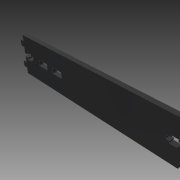
# Autodesk Inventor part: front_panel_2004_front
Saved by Autodesk Inventor 2014 (Build 180170000, 170)
## iProperties
Created: 2014-01-11
Part Number: front_panel_2004_front
Material: Generic
Document SubType Name: Modeling
Designer: buben
Density: 1 g/cm^3
Appearance: Anodized - Dark Gray
Author: buben
Autodesk Inventor part; units mm, degrees
ref_plane "YZ Plane" through (0, 0, 0) normal (1, 0, 0) x (0, 1, 0)
ref_plane "XZ Plane" through (0, 0, 0) normal (0, 1, 0) x (-1, 0, 0)
ref_plane "XY Plane" through (0, 0, 0) normal (0, 0, 1) x (1, 0, 0)
sketch "Sketch1" plane through (0, 0, 0) normal (0, 1, 0) x (-1, 0, 0)
  line L0 (0, 0) -> (220, 0)
  line L1 (220, 0) -> (220, 53.1)
  line L2 (220, 53.1) -> (0, 53.1)
  line L3 (0, 53.1) -> (0, 0)
  dimension "d0" = 53.1
  dimension "d1" = 220
  constraints: 8 end point, 2 parallel, 1 horizontal, 1 perpendicular
  measures "d0" distance of L2.end L0.start
  measures "d1" distance of L1.end L2.end
extrude "Extrusion1" add sketch "Sketch1" along normal blind 6
sketch "Sketch2" plane through (0, 6, 0) normal (0, 1, 0) x (1, 0, 0)
  line L0 (-220, 0) -> (-220, -53.1) projected
  line L1 (0, -53.1) -> (0, 0) projected
  line L2 (-220, -8.0055) -> (-224, -8.0055)
  line L3 (-226, -10.0055) -> (-226, -14.0055)
  line L4 (-224, -16.0055) -> (-220, -16.0055)
  line L5 (-220, -16.0055) -> (-220, -8.0055)
  line L6 (-220, -37.0945) -> (-224, -37.0945)
  line L7 (-226, -39.0945) -> (-226, -43.0945)
  line L8 (-224, -45.0945) -> (-220, -45.0945)
  line L9 (-220, -45.0945) -> (-220, -37.0945)
  line L10 (0, -8.0055) -> (4, -8.0055)
  line L11 (6, -10.0055) -> (6, -14.0055)
  line L12 (4, -16.0055) -> (0, -16.0055)
  line L13 (0, -16.0055) -> (0, -8.0055)
  line L14 (0, -37.0945) -> (4, -37.0945)
  line L15 (6, -39.0945) -> (6, -43.0945)
  line L16 (4, -45.0945) -> (0, -45.0945)
  line L17 (0, -45.0945) -> (0, -37.0945)
  arc A0 (-224, -8.0055) -> (-226, -10.0055) centre (-224, -10.0055) ccw
  arc A1 (-226, -14.0055) -> (-224, -16.0055) centre (-224, -14.0055) ccw
  arc A2 (-224, -37.0945) -> (-226, -39.0945) centre (-224, -39.0945) ccw
  arc A3 (-226, -43.0945) -> (-224, -45.0945) centre (-224, -43.0945) ccw
  arc A4 (4, -45.0945) -> (6, -43.0945) centre (4, -43.0945) ccw
  arc A5 (6, -39.0945) -> (4, -37.0945) centre (4, -39.0945) ccw
  arc A6 (4, -16.0055) -> (6, -14.0055) centre (4, -14.0055) ccw
  arc A7 (6, -10.0055) -> (4, -8.0055) centre (4, -10.0055) ccw
  line L18 (-222, -16.0055) -> (-222, -37.0945) construction
  point P0 (-222, -26.55)
  point P1 (-220, -26.55)
  dimension "d4" = 2
  dimension "d5" = 8
  dimension "d6" = 8
  dimension "d7" = 6
  dimension "d8" = 6
  dimension "d9" = 21.089
  constraints: 34 end point, 16 point on circle, 16 tangent, 8 centre point, 8 parallel, 7 equal radius, 6 collinear, 4 horizontal, 4 midpoint, 4 perpendicular, 4 point on line, 1 horizontal alignment
  measures "d4" radius of A0
  measures "d5" distance between parallel lines of L4 L2
  measures "d6" distance between parallel lines of L8 L6
  measures "d7" distance between parallel lines of L0 L3
  measures "d8" distance between parallel lines of L1 L11
  measures "d9" distance of L18.start L18.end
extrude "Extrusion2" add sketch "Sketch2" against normal blind 6
sketch "Sketch3" plane through (0, 6, 0) normal (0, 1, 0) x (1, 0, 0)
  line L0 (0, 0) -> (-220, 0) projected
  line L1 (-220, -16.0055) -> (-220, -37.0945) projected
  line L2 (-220, -53.1) -> (0, -53.1) projected
  line L3 (-203.7, -24.3) -> (-203.7, -28.8)
  line L4 (-220, -28.8) -> (-220, -24.3)
  line L5 (-215, -21.8) -> (-207.7, -21.8)
  line L6 (-207.7, -31.3) -> (-215, -31.3)
  line L7 (-220, -24.3) -> (-215, -24.3)
  line L8 (-207.7, -24.3) -> (-203.7, -24.3)
  line L9 (-203.7, -28.8) -> (-207.7, -28.8)
  line L10 (-215, -28.8) -> (-220, -28.8)
  line L11 (-207.7, -21.8) -> (-207.7, -24.3)
  line L12 (-207.7, -28.8) -> (-207.7, -31.3)
  line L13 (-215, -31.3) -> (-215, -28.8)
  line L14 (-215, -24.3) -> (-215, -21.8)
  line L15 (-110, 0) -> (-110, -53.1) construction
  line L16 (-16.3, -24.3) -> (-16.3, -28.8)
  line L17 (0, -28.8) -> (0, -24.3)
  line L18 (-5, -21.8) -> (-12.3, -21.8)
  line L19 (-12.3, -31.3) -> (-5, -31.3)
  line L20 (0, -24.3) -> (-5, -24.3)
  line L21 (-12.3, -24.3) -> (-16.3, -24.3)
  line L22 (-16.3, -28.8) -> (-12.3, -28.8)
  line L23 (-5, -28.8) -> (0, -28.8)
  line L24 (-12.3, -21.8) -> (-12.3, -24.3)
  line L25 (-12.3, -28.8) -> (-12.3, -31.3)
  line L26 (-5, -31.3) -> (-5, -28.8)
  line L27 (-5, -24.3) -> (-5, -21.8)
  point P0 (-203.7, -26.55)
  point P1 (-220, -26.55)
  point P2 (-16.3, -26.55)
  point P3 (0, -26.55)
  dimension "d12" = 4.5
  dimension "d13" = 2.5
  dimension "d14" = 2.5
  dimension "d15" = 5
  dimension "d16" = 4
  dimension "d17" = 7.3
  constraints: 50 end point, 14 symmetric about line, 10 parallel, 5 collinear, 4 midpoint, 4 perpendicular, 3 horizontal, 1 horizontal alignment
  measures "d12" distance of L3.start L3.end
  measures "d13" distance of L5.end L8.start
  measures "d14" distance of L9.end L6.start
  measures "d15" distance of L10.start L4.start
  measures "d16" distance of L3.end L9.end
  measures "d17" distance of L6.start L6.end
extrude "Extrusion3" cut sketch "Sketch3" against normal blind 6
sketch "Sketch4" plane through (0, 0, 0) normal (0, -1, 0) x (1, 0, 0)
  line L0 (-203.7, 28.8) -> (-203.7, 24.3) projected
  line L1 (-190.7, 30.55) -> (-177.7, 30.55)
  line L2 (-176.7, 29.55) -> (-176.7, 23.55)
  line L3 (-177.7, 22.55) -> (-190.7, 22.55)
  line L4 (-191.7, 23.55) -> (-191.7, 29.55)
  line L5 (-165.7, 30.55) -> (-152.7, 30.55)
  line L6 (-151.7, 29.55) -> (-151.7, 23.55)
  line L7 (-152.7, 22.55) -> (-165.7, 22.55)
  line L8 (-166.7, 23.55) -> (-166.7, 29.55)
  arc A0 (-190.7, 30.55) -> (-191.7, 29.55) centre (-190.7, 29.55) ccw
  arc A1 (-176.7, 29.55) -> (-177.7, 30.55) centre (-177.7, 29.55) ccw
  arc A2 (-177.7, 22.55) -> (-176.7, 23.55) centre (-177.7, 23.55) ccw
  arc A3 (-191.7, 23.55) -> (-190.7, 22.55) centre (-190.7, 23.55) ccw
  arc A4 (-165.7, 30.55) -> (-166.7, 29.55) centre (-165.7, 29.55) ccw
  arc A5 (-151.7, 29.55) -> (-152.7, 30.55) centre (-152.7, 29.55) ccw
  arc A6 (-152.7, 22.55) -> (-151.7, 23.55) centre (-152.7, 23.55) ccw
  arc A7 (-166.7, 23.55) -> (-165.7, 22.55) centre (-165.7, 23.55) ccw
  point P0 (-203.7, 26.55)
  point P1 (-191.7, 26.55)
  dimension "d20" = 1
  dimension "d21" = 15
  dimension "d22" = 15
  dimension "d23" = 8
  dimension "d24" = 10
  dimension "d25" = 12
  constraints: 16 end point, 16 point on circle, 16 tangent, 8 centre point, 7 equal radius, 4 parallel, 2 collinear, 2 horizontal, 2 midpoint, 2 perpendicular, 1 horizontal alignment
  measures "d20" radius of A0
  measures "d21" distance between parallel lines of L2 L4
  measures "d22" distance between parallel lines of L6 L8
  measures "d23" distance between parallel lines of L3 L1
  measures "d24" distance between parallel lines of L8 L2
  measures "d25" distance between parallel lines of L0 L4
extrude "Extrusion4" cut sketch "Sketch4" against normal through all
sketch "Sketch6" plane through (0, 6, 0) normal (0, 1, 0) x (1, 0, 0)
  line L0 (-220, -53.1) -> (0, -53.1) projected
  line L1 (0, -53.1) -> (0, -45.0945) projected
  line L2 (-50, -37.1) -> (-10, -37.1) construction
  line L3 (-10, -37.1) -> (-10, -47.1) construction
  line L4 (-10, -47.1) -> (-50, -47.1) construction
  line L5 (-50, -47.1) -> (-50, -37.1) construction
  spline S0 degree 2 poles (-43.1283, -39.4018) (-43.1283, -40.2833) (-43.8661, -40.7828) knots 0 0 0 1 1 1
  spline S1 degree 2 poles (-43.8661, -40.7828) (-44.16, -40.9787) (-44.5518, -40.9787) knots 0 0 0 1 1 1
  line L6 (-44.5518, -40.9787) -> (-45.9035, -40.9787)
  spline S2 degree 2 poles (-45.9035, -40.9787) (-46.07, -40.9787) (-46.07, -40.8514) knots 0 0 0 1 1 1
  spline S3 degree 2 poles (-46.07, -40.8514) (-46.07, -40.7273) (-45.9035, -40.7273) knots 0 0 0 1 1 1
  line L7 (-45.9035, -40.7273) -> (-45.6912, -40.7273)
  line L8 (-45.6912, -40.7273) -> (-45.6912, -37.7301)
  line L9 (-45.6912, -37.7301) -> (-45.9035, -37.7301)
  spline S4 degree 2 poles (-45.9035, -37.7301) (-46.07, -37.7301) (-46.07, -37.6028) knots 0 0 0 1 1 1
  spline S5 degree 2 poles (-46.07, -37.6028) (-46.07, -37.4787) (-45.9035, -37.4787) knots 0 0 0 1 1 1
  line L10 (-45.9035, -37.4787) -> (-44.5518, -37.4787)
  spline S6 degree 2 poles (-44.5518, -37.4787) (-43.9282, -37.4787) (-43.5723, -37.9097) knots 0 0 0 1 1 1
  spline S7 degree 2 poles (-43.5723, -37.9097) (-43.1283, -38.4484) (-43.1283, -39.0557) knots 0 0 0 1 1 1
  line L11 (-43.1283, -39.0557) -> (-43.1283, -39.4018)
  line L12 (-43.3797, -39.4573) -> (-43.3797, -39.0002)
  spline S8 degree 2 poles (-43.3797, -39.0002) (-43.3797, -38.7684) (-43.4548, -38.5855) knots 0 0 0 1 1 1
  spline S9 degree 2 poles (-43.4548, -38.5855) (-43.5625, -38.3178) (-43.7584, -38.0795) knots 0 0 0 1 1 1
  spline S10 degree 2 poles (-43.7584, -38.0795) (-44.0457, -37.7301) (-44.5289, -37.7301) knots 0 0 0 1 1 1
  line L13 (-44.5289, -37.7301) -> (-45.4398, -37.7301)
  line L14 (-45.4398, -37.7301) -> (-45.4398, -40.7273)
  line L15 (-45.4398, -40.7273) -> (-44.5289, -40.7273)
  spline S11 degree 2 poles (-44.5289, -40.7273) (-44.2155, -40.7273) (-43.9314, -40.5184) knots 0 0 0 1 1 1
  spline S12 degree 2 poles (-43.9314, -40.5184) (-43.6604, -40.3225) (-43.5168, -40.0254) knots 0 0 0 1 1 1
  spline S13 degree 2 poles (-43.5168, -40.0254) (-43.3797, -39.7381) (-43.3797, -39.4573) knots 0 0 0 1 1 1
  spline S14 degree 2 poles (-39.6642, -40.5674) (-39.6642, -40.6163) (-39.7132, -40.6686) knots 0 0 0 1 1 1
  spline S15 degree 2 poles (-39.7132, -40.6686) (-39.896, -40.8547) (-40.3041, -40.9755) knots 0 0 0 1 1 1
  spline S16 degree 2 poles (-40.3041, -40.9755) (-40.66, -41.0767) (-40.9734, -41.0767) knots 0 0 0 1 1 1
  spline S17 degree 2 poles (-40.9734, -41.0767) (-41.6035, -41.0767) (-42.0378, -40.6686) knots 0 0 0 1 1 1
  spline S18 degree 2 poles (-42.0378, -40.6686) (-42.4851, -40.2539) (-42.4851, -39.6303) knots 0 0 0 1 1 1
  spline S19 degree 2 poles (-42.4851, -39.6303) (-42.4851, -39.0557) (-42.0639, -38.6704) knots 0 0 0 1 1 1
  spline S20 degree 2 poles (-42.0639, -38.6704) (-41.6525, -38.2982) (-41.0779, -38.2982) knots 0 0 0 1 1 1
  spline S21 degree 2 poles (-41.0779, -38.2982) (-40.4445, -38.2982) (-39.6642, -39.1112) (-39.6707, -39.7446) knots 0 0 0 1 2 2 2
  line L16 (-39.6707, -39.7446) -> (-42.2304, -39.7446)
  spline S22 degree 2 poles (-42.2304, -39.7446) (-42.1651, -40.2409) (-41.4762, -40.8253) (-40.9734, -40.8253) knots 0 0 0 1 2 2 2
  spline S23 degree 2 poles (-40.9734, -40.8253) (-40.3139, -40.8253) (-39.8829, -40.489) knots 0 0 0 1 1 1
  spline S24 degree 2 poles (-39.8829, -40.489) (-39.8242, -40.4433) (-39.785, -40.4433) knots 0 0 0 1 1 1
  spline S25 degree 2 poles (-39.785, -40.4433) (-39.6642, -40.4433) (-39.6642, -40.5674) knots 0 0 0 1 1 1
  spline S26 degree 2 poles (-39.9254, -39.4899) (-40.0005, -39.0655) (-40.6437, -38.5529) (-41.0746, -38.5529) knots 0 0 0 1 2 2 2
  spline S27 degree 2 poles (-41.0746, -38.5529) (-41.5121, -38.5529) (-42.1488, -39.0622) (-42.2271, -39.4899) knots 0 0 0 1 2 2 2
  line L17 (-42.2271, -39.4899) -> (-39.9254, -39.4899)
  spline S28 degree 2 poles (-36.1348, -40.2572) (-36.1348, -40.6751) (-36.5527, -40.8971) knots 0 0 0 1 1 1
  spline S29 degree 2 poles (-36.5527, -40.8971) (-36.8923, -41.0767) (-37.3461, -41.0767) knots 0 0 0 1 1 1
  spline S30 degree 2 poles (-37.3461, -41.0767) (-37.9403, -41.0767) (-38.319, -40.7763) knots 0 0 0 1 1 1
  spline S31 degree 2 poles (-38.319, -40.7763) (-38.319, -40.9232) (-38.3713, -40.9591) knots 0 0 0 1 1 1
  spline S32 degree 2 poles (-38.3713, -40.9591) (-38.4072, -40.9787) (-38.4431, -40.9787) knots 0 0 0 1 1 1
  spline S33 degree 2 poles (-38.4431, -40.9787) (-38.5704, -40.9787) (-38.5704, -40.8122) knots 0 0 0 1 1 1
  line L18 (-38.5704, -40.8122) -> (-38.5704, -40.2931)
  spline S34 degree 2 poles (-38.5704, -40.2931) (-38.5704, -40.1266) (-38.4431, -40.1266) knots 0 0 0 1 1 1
  spline S35 degree 2 poles (-38.4431, -40.1266) (-38.3158, -40.1266) (-38.3158, -40.2637) knots 0 0 0 1 1 1
  spline S36 degree 2 poles (-38.3158, -40.2637) (-38.3158, -40.5641) (-37.9109, -40.7306) knots 0 0 0 1 1 1
  spline S37 degree 2 poles (-37.9109, -40.7306) (-37.6856, -40.8253) (-37.3526, -40.8253) knots 0 0 0 1 1 1
  spline S38 degree 2 poles (-37.3526, -40.8253) (-37.0163, -40.8253) (-36.7486, -40.7077) knots 0 0 0 1 1 1
  spline S39 degree 2 poles (-36.7486, -40.7077) (-36.3862, -40.5543) (-36.3862, -40.2572) knots 0 0 0 1 1 1
  spline S40 degree 2 poles (-36.3862, -40.2572) (-36.3862, -39.7936) (-37.3396, -39.6956) knots 0 0 0 1 1 1
  spline S41 degree 2 poles (-37.3396, -39.6956) (-37.715, -39.6564) (-37.8783, -39.6107) knots 0 0 0 1 1 1
  spline S42 degree 2 poles (-37.8783, -39.6107) (-38.1884, -39.5258) (-38.3288, -39.3365) knots 0 0 0 1 1 1
  spline S43 degree 2 poles (-38.3288, -39.3365) (-38.4431, -39.1798) (-38.4431, -39.0002) knots 0 0 0 1 1 1
  spline S44 degree 2 poles (-38.4431, -39.0002) (-38.4431, -38.6443) (-38.0644, -38.4517) knots 0 0 0 1 1 1
  spline S45 degree 2 poles (-38.0644, -38.4517) (-37.7607, -38.2982) (-37.3689, -38.2982) knots 0 0 0 1 1 1
  spline S46 degree 2 poles (-37.3689, -38.2982) (-36.8498, -38.2982) (-36.5233, -38.5496) knots 0 0 0 1 1 1
  spline S47 degree 2 poles (-36.5233, -38.5496) (-36.5233, -38.3864) (-36.396, -38.3864) knots 0 0 0 1 1 1
  spline S48 degree 2 poles (-36.396, -38.3864) (-36.2687, -38.3864) (-36.2687, -38.5562) knots 0 0 0 1 1 1
  line L19 (-36.2687, -38.5562) -> (-36.2687, -38.9904)
  spline S49 degree 2 poles (-36.2687, -38.9904) (-36.2687, -39.1569) (-36.396, -39.1569) knots 0 0 0 1 1 1
  spline S50 degree 2 poles (-36.396, -39.1569) (-36.5103, -39.1569) (-36.5233, -39.0165) knots 0 0 0 1 1 1
  spline S51 degree 2 poles (-36.5233, -39.0165) (-36.5396, -38.8369) (-36.7094, -38.7194) knots 0 0 0 1 1 1
  spline S52 degree 2 poles (-36.7094, -38.7194) (-36.951, -38.5529) (-37.3559, -38.5529) knots 0 0 0 1 1 1
  spline S53 degree 2 poles (-37.3559, -38.5529) (-37.7803, -38.5529) (-38.0121, -38.7227) knots 0 0 0 1 1 1
  spline S54 degree 2 poles (-38.0121, -38.7227) (-38.1884, -38.8533) (-38.1884, -39.01) knots 0 0 0 1 1 1
  spline S55 degree 2 poles (-38.1884, -39.01) (-38.1884, -39.1896) (-37.9795, -39.3104) knots 0 0 0 1 1 1
  spline S56 degree 2 poles (-37.9795, -39.3104) (-37.8326, -39.392) (-37.4342, -39.4377) knots 0 0 0 1 1 1
  spline S57 degree 2 poles (-37.4342, -39.4377) (-36.9053, -39.4965) (-36.7094, -39.565) knots 0 0 0 1 1 1
  spline S58 degree 2 poles (-36.7094, -39.565) (-36.1348, -39.774) (-36.1348, -40.2572) knots 0 0 0 1 1 1
  spline S59 degree 2 poles (-32.3867, -40.8514) (-32.3867, -40.9787) (-32.5564, -40.9787) knots 0 0 0 1 1 1
  line L20 (-32.5564, -40.9787) -> (-34.7831, -40.9787)
  spline S60 degree 2 poles (-34.7831, -40.9787) (-34.9496, -40.9787) (-34.9496, -40.8514) knots 0 0 0 1 1 1
  spline S61 degree 2 poles (-34.9496, -40.8514) (-34.9496, -40.7273) (-34.7831, -40.7273) knots 0 0 0 1 1 1
  line L21 (-34.7831, -40.7273) -> (-33.7938, -40.7273)
  line L22 (-33.7938, -40.7273) -> (-33.7938, -38.6443)
  line L23 (-33.7938, -38.6443) -> (-34.5285, -38.6443)
  spline S62 degree 2 poles (-34.5285, -38.6443) (-34.6982, -38.6443) (-34.6982, -38.517) knots 0 0 0 1 1 1
  spline S63 degree 2 poles (-34.6982, -38.517) (-34.6982, -38.3896) (-34.5285, -38.3896) knots 0 0 0 1 1 1
  line L24 (-34.5285, -38.3896) -> (-33.5424, -38.3896)
  line L25 (-33.5424, -38.3896) -> (-33.5424, -40.7273)
  line L26 (-33.5424, -40.7273) -> (-32.5564, -40.7273)
  spline S64 degree 2 poles (-32.5564, -40.7273) (-32.3867, -40.7273) (-32.3867, -40.8514) knots 0 0 0 1 1 1
  line L27 (-33.549, -37.7497) -> (-33.9212, -37.7497)
  line L28 (-33.9212, -37.7497) -> (-33.9212, -37.1)
  line L29 (-33.9212, -37.1) -> (-33.549, -37.1)
  line L30 (-33.549, -37.1) -> (-33.549, -37.7497)
  spline S65 degree 2 poles (-28.3969, -38.517) (-28.3969, -38.6443) (-28.5634, -38.6443) knots 0 0 0 1 1 1
  line L31 (-28.5634, -38.6443) -> (-28.903, -38.6443)
  line L32 (-28.903, -38.6443) -> (-28.903, -41.1518)
  spline S66 degree 2 poles (-28.903, -41.1518) (-28.903, -41.4032) (-29.0107, -41.5991) knots 0 0 0 1 1 1
  spline S67 degree 2 poles (-29.0107, -41.5991) (-29.1772, -41.906) (-29.556, -42.0725) knots 0 0 0 1 1 1
  spline S68 degree 2 poles (-29.556, -42.0725) (-29.6931, -42.1313) (-29.9249, -42.1313) knots 0 0 0 1 1 1
  line L33 (-29.9249, -42.1313) -> (-30.6367, -42.1313)
  spline S69 degree 2 poles (-30.6367, -42.1313) (-30.8032, -42.1313) (-30.8032, -42.0039) knots 0 0 0 1 1 1
  spline S70 degree 2 poles (-30.8032, -42.0039) (-30.8032, -41.8766) (-30.6367, -41.8766) knots 0 0 0 1 1 1
  line L34 (-30.6367, -41.8766) -> (-29.9151, -41.8799)
  spline S71 degree 2 poles (-29.9151, -41.8799) (-29.458, -41.8831) (-29.2197, -41.4358) knots 0 0 0 1 1 1
  spline S72 degree 2 poles (-29.2197, -41.4358) (-29.1544, -41.3118) (-29.1544, -41.1159) knots 0 0 0 1 1 1
  line L35 (-29.1544, -41.1159) -> (-29.1544, -40.3617)
  spline S73 degree 2 poles (-29.1544, -40.3617) (-29.5592, -40.9167) (-30.1959, -40.9167) knots 0 0 0 1 1 1
  spline S74 degree 2 poles (-30.1959, -40.9167) (-30.7281, -40.9167) (-31.097, -40.5249) knots 0 0 0 1 1 1
  spline S75 degree 2 poles (-31.097, -40.5249) (-31.4627, -40.1429) (-31.4627, -39.6075) knots 0 0 0 1 1 1
  spline S76 degree 2 poles (-31.4627, -39.6075) (-31.4627, -39.0688) (-30.7281, -38.2982) (-30.1959, -38.2982) knots 0 0 0 1 2 2 2
  spline S77 degree 2 poles (-30.1959, -38.2982) (-29.5592, -38.2982) (-29.1544, -38.85) knots 0 0 0 1 1 1
  line L36 (-29.1544, -38.85) -> (-29.1544, -38.3896)
  line L37 (-29.1544, -38.3896) -> (-28.5634, -38.3896)
  spline S78 degree 2 poles (-28.5634, -38.3896) (-28.3969, -38.3896) (-28.3969, -38.517) knots 0 0 0 1 1 1
  spline S79 degree 2 poles (-29.1544, -39.6075) (-29.1544, -39.17) (-29.7486, -38.5529) (-30.1828, -38.5529) knots 0 0 0 1 2 2 2
  spline S80 degree 2 poles (-30.1828, -38.5529) (-30.6171, -38.5529) (-31.208, -39.1732) (-31.208, -39.6075) knots 0 0 0 1 2 2 2
  spline S81 degree 2 poles (-31.208, -39.6075) (-31.208, -40.0417) (-30.6171, -40.662) (-30.1828, -40.662) knots 0 0 0 1 2 2 2
  spline S82 degree 2 poles (-30.1828, -40.662) (-29.7486, -40.662) (-29.1544, -40.0417) (-29.1544, -39.6075) knots 0 0 0 1 2 2 2
  spline S83 degree 2 poles (-24.8414, -40.8514) (-24.8414, -40.9787) (-25.0079, -40.9787) knots 0 0 0 1 1 1
  line L38 (-25.0079, -40.9787) -> (-25.6805, -40.9787)
  spline S84 degree 2 poles (-25.6805, -40.9787) (-25.8503, -40.9787) (-25.8503, -40.8514) knots 0 0 0 1 1 1
  spline S85 degree 2 poles (-25.8503, -40.8514) (-25.8503, -40.7273) (-25.6805, -40.7273) knots 0 0 0 1 1 1
  line L39 (-25.6805, -40.7273) -> (-25.4715, -40.7273)
  line L40 (-25.4715, -40.7273) -> (-25.4715, -39.1863)
  spline S86 degree 2 poles (-25.4715, -39.1863) (-25.4715, -38.8924) (-25.687, -38.7161) knots 0 0 0 1 1 1
  spline S87 degree 2 poles (-25.687, -38.7161) (-25.8862, -38.5529) (-26.1866, -38.5529) knots 0 0 0 1 1 1
  spline S88 degree 2 poles (-26.1866, -38.5529) (-26.4902, -38.5529) (-26.7285, -38.7292) knots 0 0 0 1 1 1
  spline S89 degree 2 poles (-26.7285, -38.7292) (-26.8657, -38.8304) (-27.1367, -39.1504) knots 0 0 0 1 1 1
  line L41 (-27.1367, -39.1504) -> (-27.1367, -40.7273)
  line L42 (-27.1367, -40.7273) -> (-26.8526, -40.7273)
  spline S90 degree 2 poles (-26.8526, -40.7273) (-26.6861, -40.7273) (-26.6861, -40.8514) knots 0 0 0 1 1 1
  spline S91 degree 2 poles (-26.6861, -40.8514) (-26.6861, -40.9787) (-26.8526, -40.9787) knots 0 0 0 1 1 1
  line L43 (-26.8526, -40.9787) -> (-27.6721, -40.9787)
  spline S92 degree 2 poles (-27.6721, -40.9787) (-27.8386, -40.9787) (-27.8386, -40.8514) knots 0 0 0 1 1 1
  spline S93 degree 2 poles (-27.8386, -40.8514) (-27.8386, -40.7273) (-27.6721, -40.7273) knots 0 0 0 1 1 1
  line L44 (-27.6721, -40.7273) -> (-27.3881, -40.7273)
  line L45 (-27.3881, -40.7273) -> (-27.3881, -38.6443)
  line L46 (-27.3881, -38.6443) -> (-27.6003, -38.6443)
  spline S94 degree 2 poles (-27.6003, -38.6443) (-27.7668, -38.6443) (-27.7668, -38.517) knots 0 0 0 1 1 1
  spline S95 degree 2 poles (-27.7668, -38.517) (-27.7668, -38.3896) (-27.6003, -38.3896) knots 0 0 0 1 1 1
  line L47 (-27.6003, -38.3896) -> (-27.1367, -38.3896)
  line L48 (-27.1367, -38.3896) -> (-27.1367, -38.7684)
  spline S96 degree 2 poles (-27.1367, -38.7684) (-26.673, -38.2982) (-26.1833, -38.2982) knots 0 0 0 1 1 1
  spline S97 degree 2 poles (-26.1833, -38.2982) (-25.6283, -38.2982) (-25.354, -38.7161) knots 0 0 0 1 1 1
  spline S98 degree 2 poles (-25.354, -38.7161) (-25.2201, -38.9251) (-25.2201, -39.1438) knots 0 0 0 1 1 1
  line L49 (-25.2201, -39.1438) -> (-25.2201, -40.7273)
  line L50 (-25.2201, -40.7273) -> (-25.0079, -40.7273)
  spline S99 degree 2 poles (-25.0079, -40.7273) (-24.8414, -40.7273) (-24.8414, -40.8514) knots 0 0 0 1 1 1
  spline S100 degree 2 poles (-17.4855, -39.676) (-17.4855, -40.2441) (-17.8643, -40.6555) knots 0 0 0 1 1 1
  spline S101 degree 2 poles (-17.8643, -40.6555) (-18.2528, -41.0767) (-18.8209, -41.0767) knots 0 0 0 1 1 1
  spline S102 degree 2 poles (-18.8209, -41.0767) (-19.4771, -41.0767) (-19.9179, -40.4857) knots 0 0 0 1 1 1
  line L51 (-19.9179, -40.4857) -> (-19.9179, -40.9787)
  line L52 (-19.9179, -40.9787) -> (-20.5089, -40.9787)
  spline S103 degree 2 poles (-20.5089, -40.9787) (-20.6754, -40.9787) (-20.6754, -40.8514) knots 0 0 0 1 1 1
  spline S104 degree 2 poles (-20.6754, -40.8514) (-20.6754, -40.7273) (-20.5089, -40.7273) knots 0 0 0 1 1 1
  line L53 (-20.5089, -40.7273) -> (-20.1693, -40.7273)
  line L54 (-20.1693, -40.7273) -> (-20.1693, -37.4787)
  line L55 (-20.1693, -37.4787) -> (-20.5089, -37.4787)
  spline S105 degree 2 poles (-20.5089, -37.4787) (-20.6754, -37.4787) (-20.6754, -37.3514) knots 0 0 0 1 1 1
  spline S106 degree 2 poles (-20.6754, -37.3514) (-20.6754, -37.2241) (-20.5089, -37.2241) knots 0 0 0 1 1 1
  line L56 (-20.5089, -37.2241) -> (-19.9179, -37.2241)
  line L57 (-19.9179, -37.2241) -> (-19.9179, -38.8892)
  spline S107 degree 2 poles (-19.9179, -38.8892) (-19.4641, -38.2982) (-18.8209, -38.2982) knots 0 0 0 1 1 1
  spline S108 degree 2 poles (-18.8209, -38.2982) (-18.2528, -38.2982) (-17.4855, -39.1047) (-17.4855, -39.676) knots 0 0 0 1 2 2 2
  spline S109 degree 2 poles (-17.7369, -39.6891) (-17.7369, -39.2287) (-18.0471, -38.8924) knots 0 0 0 1 1 1
  spline S110 degree 2 poles (-18.0471, -38.8924) (-18.3671, -38.5529) (-18.8242, -38.5529) knots 0 0 0 1 1 1
  spline S111 degree 2 poles (-18.8242, -38.5529) (-19.2845, -38.5529) (-19.9146, -39.2287) (-19.9146, -39.6891) knots 0 0 0 1 2 2 2
  spline S112 degree 2 poles (-19.9146, -39.6891) (-19.9146, -40.1494) (-19.2845, -40.8253) (-18.8242, -40.8253) knots 0 0 0 1 2 2 2
  spline S113 degree 2 poles (-18.8242, -40.8253) (-18.3671, -40.8253) (-18.0471, -40.4857) knots 0 0 0 1 1 1
  spline S114 degree 2 poles (-18.0471, -40.4857) (-17.7369, -40.1494) (-17.7369, -39.6891) knots 0 0 0 1 1 1
  spline S115 degree 2 poles (-13.6199, -38.517) (-13.6199, -38.6051) (-13.6982, -38.6313) knots 0 0 0 1 1 1
  spline S116 degree 2 poles (-13.6982, -38.6313) (-13.7276, -38.6443) (-13.8647, -38.6443) knots 0 0 0 1 1 1
  line L58 (-13.8647, -38.6443) -> (-15.4515, -41.8799)
  line L59 (-15.4515, -41.8799) -> (-15.0597, -41.8799)
  spline S117 degree 2 poles (-15.0597, -41.8799) (-14.8932, -41.8799) (-14.8932, -42.0039) knots 0 0 0 1 1 1
  spline S118 degree 2 poles (-14.8932, -42.0039) (-14.8932, -42.1313) (-15.0597, -42.1313) knots 0 0 0 1 1 1
  line L60 (-15.0597, -42.1313) -> (-16.5093, -42.1313)
  spline S119 degree 2 poles (-16.5093, -42.1313) (-16.6758, -42.1313) (-16.6758, -42.0039) knots 0 0 0 1 1 1
  spline S120 degree 2 poles (-16.6758, -42.0039) (-16.6758, -41.8799) (-16.5093, -41.8799) knots 0 0 0 1 1 1
  line L61 (-16.5093, -41.8799) -> (-15.7225, -41.8799)
  line L62 (-15.7225, -41.8799) -> (-15.2785, -40.9787)
  line L63 (-15.2785, -40.9787) -> (-16.4473, -38.6443)
  line L64 (-16.4473, -38.6443) -> (-16.5224, -38.6443)
  spline S121 degree 2 poles (-16.5224, -38.6443) (-16.6889, -38.6443) (-16.6889, -38.517) knots 0 0 0 1 1 1
  spline S122 degree 2 poles (-16.6889, -38.517) (-16.6889, -38.4354) (-16.6171, -38.4027) knots 0 0 0 1 1 1
  spline S123 degree 2 poles (-16.6171, -38.4027) (-16.5877, -38.3896) (-16.5224, -38.3896) knots 0 0 0 1 1 1
  line L65 (-16.5224, -38.3896) -> (-15.8335, -38.3896)
  spline S124 degree 2 poles (-15.8335, -38.3896) (-15.667, -38.3896) (-15.667, -38.517) knots 0 0 0 1 1 1
  spline S125 degree 2 poles (-15.667, -38.517) (-15.667, -38.6443) (-15.8335, -38.6443) knots 0 0 0 1 1 1
  line L66 (-15.8335, -38.6443) -> (-16.173, -38.6443)
  line L67 (-16.173, -38.6443) -> (-15.1413, -40.7012)
  line L68 (-15.1413, -40.7012) -> (-14.1357, -38.6443)
  line L69 (-14.1357, -38.6443) -> (-14.4753, -38.6443)
  spline S126 degree 2 poles (-14.4753, -38.6443) (-14.6418, -38.6443) (-14.6418, -38.517) knots 0 0 0 1 1 1
  spline S127 degree 2 poles (-14.6418, -38.517) (-14.6418, -38.3896) (-14.4753, -38.3896) knots 0 0 0 1 1 1
  line L70 (-14.4753, -38.3896) -> (-13.7896, -38.3896)
  spline S128 degree 2 poles (-13.7896, -38.3896) (-13.6199, -38.3896) (-13.6199, -38.517) knots 0 0 0 1 1 1
  spline S129 degree 2 poles (-47.2257, -46.6443) (-47.2257, -46.7717) (-47.3923, -46.7717) knots 0 0 0 1 1 1
  line L71 (-47.3923, -46.7717) -> (-49.3675, -46.7717)
  spline S130 degree 2 poles (-49.3675, -46.7717) (-49.534, -46.7717) (-49.534, -46.6443) knots 0 0 0 1 1 1
  spline S131 degree 2 poles (-49.534, -46.6443) (-49.534, -46.5203) (-49.3675, -46.5203) knots 0 0 0 1 1 1
  line L72 (-49.3675, -46.5203) -> (-48.5056, -46.5203)
  line L73 (-48.5056, -46.5203) -> (-48.5056, -43.5231)
  line L74 (-48.5056, -43.5231) -> (-49.3675, -43.5231)
  spline S132 degree 2 poles (-49.3675, -43.5231) (-49.534, -43.5231) (-49.534, -43.3957) knots 0 0 0 1 1 1
  spline S133 degree 2 poles (-49.534, -43.3957) (-49.534, -43.2717) (-49.3675, -43.2717) knots 0 0 0 1 1 1
  line L75 (-49.3675, -43.2717) -> (-47.3923, -43.2717)
  spline S134 degree 2 poles (-47.3923, -43.2717) (-47.2257, -43.2717) (-47.2257, -43.3957) knots 0 0 0 1 1 1
  spline S135 degree 2 poles (-47.2257, -43.3957) (-47.2257, -43.5231) (-47.3923, -43.5231) knots 0 0 0 1 1 1
  line L76 (-47.3923, -43.5231) -> (-48.2542, -43.5231)
  line L77 (-48.2542, -43.5231) -> (-48.2542, -46.5203)
  line L78 (-48.2542, -46.5203) -> (-47.3923, -46.5203)
  spline S136 degree 2 poles (-47.3923, -46.5203) (-47.2257, -46.5203) (-47.2257, -46.6443) knots 0 0 0 1 1 1
  spline S137 degree 2 poles (-43.0466, -44.3099) (-43.0466, -44.4372) (-43.2132, -44.4372) knots 0 0 0 1 1 1
  line L79 (-43.2132, -44.4372) -> (-43.4678, -44.4372)
  line L80 (-43.4678, -44.4372) -> (-44.4865, -46.7717)
  line L81 (-44.4865, -46.7717) -> (-44.9109, -46.7717)
  line L82 (-44.9109, -46.7717) -> (-45.9426, -44.4372)
  line L83 (-45.9426, -44.4372) -> (-46.2006, -44.4372)
  spline S138 degree 2 poles (-46.2006, -44.4372) (-46.3671, -44.4372) (-46.3671, -44.3099) knots 0 0 0 1 1 1
  spline S139 degree 2 poles (-46.3671, -44.3099) (-46.3671, -44.1826) (-46.2006, -44.1826) knots 0 0 0 1 1 1
  line L84 (-46.2006, -44.1826) -> (-45.257, -44.1826)
  spline S140 degree 2 poles (-45.257, -44.1826) (-45.0905, -44.1826) (-45.0905, -44.3099) knots 0 0 0 1 1 1
  spline S141 degree 2 poles (-45.0905, -44.3099) (-45.0905, -44.4372) (-45.257, -44.4372) knots 0 0 0 1 1 1
  line L85 (-45.257, -44.4372) -> (-45.6716, -44.4372)
  line L86 (-45.6716, -44.4372) -> (-44.7509, -46.5203)
  line L87 (-44.7509, -46.5203) -> (-44.6465, -46.5203)
  line L88 (-44.6465, -46.5203) -> (-43.7388, -44.4372)
  line L89 (-43.7388, -44.4372) -> (-44.16, -44.4372)
  spline S142 degree 2 poles (-44.16, -44.4372) (-44.3265, -44.4372) (-44.3265, -44.3099) knots 0 0 0 1 1 1
  spline S143 degree 2 poles (-44.3265, -44.3099) (-44.3265, -44.1826) (-44.16, -44.1826) knots 0 0 0 1 1 1
  line L90 (-44.16, -44.1826) -> (-43.2132, -44.1826)
  spline S144 degree 2 poles (-43.2132, -44.1826) (-43.0466, -44.1826) (-43.0466, -44.3099) knots 0 0 0 1 1 1
  spline S145 degree 2 poles (-39.625, -45.482) (-39.625, -46.0632) (-40.4445, -46.8696) (-41.0289, -46.8696) knots 0 0 0 1 2 2 2
  spline S146 degree 2 poles (-41.0289, -46.8696) (-41.6101, -46.8696) (-42.4328, -46.0664) (-42.4328, -45.482) knots 0 0 0 1 2 2 2
  spline S147 degree 2 poles (-42.4328, -45.482) (-42.4328, -44.8976) (-41.6101, -44.0911) (-41.0289, -44.0911) knots 0 0 0 1 2 2 2
  spline S148 degree 2 poles (-41.0289, -44.0911) (-40.4445, -44.0911) (-39.625, -44.8976) (-39.625, -45.482) knots 0 0 0 1 2 2 2
  spline S149 degree 2 poles (-39.8797, -45.482) (-39.8797, -45.0021) (-40.5522, -44.3458) (-41.0289, -44.3458) knots 0 0 0 1 2 2 2
  spline S150 degree 2 poles (-41.0289, -44.3458) (-41.5089, -44.3458) (-42.1814, -45.0053) (-42.1814, -45.482) knots 0 0 0 1 2 2 2
  spline S151 degree 2 poles (-42.1814, -45.482) (-42.1814, -45.9587) (-41.5056, -46.6182) (-41.0289, -46.6182) knots 0 0 0 1 2 2 2
  spline S152 degree 2 poles (-41.0289, -46.6182) (-40.5522, -46.6182) (-39.8797, -45.9587) (-39.8797, -45.482) knots 0 0 0 1 2 2 2
  spline S153 degree 2 poles (-32.3899, -45.8314) (-32.3899, -46.3244) (-32.7915, -46.6117) knots 0 0 0 1 1 1
  spline S154 degree 2 poles (-32.7915, -46.6117) (-33.1507, -46.8696) (-33.6632, -46.8696) knots 0 0 0 1 1 1
  spline S155 degree 2 poles (-33.6632, -46.8696) (-34.3195, -46.8696) (-34.7113, -46.4615) knots 0 0 0 1 1 1
  line L91 (-34.7113, -46.4615) -> (-34.7113, -46.6051)
  spline S156 degree 2 poles (-34.7113, -46.6051) (-34.7113, -46.7717) (-34.8354, -46.7717) knots 0 0 0 1 1 1
  spline S157 degree 2 poles (-34.8354, -46.7717) (-34.9627, -46.7717) (-34.9627, -46.6051) knots 0 0 0 1 1 1
  line L92 (-34.9627, -46.6051) -> (-34.9627, -45.9097)
  spline S158 degree 2 poles (-34.9627, -45.9097) (-34.9627, -45.7399) (-34.8354, -45.7399) knots 0 0 0 1 1 1
  spline S159 degree 2 poles (-34.8354, -45.7399) (-34.7211, -45.7399) (-34.7113, -45.8934) knots 0 0 0 1 1 1
  spline S160 degree 2 poles (-34.7113, -45.8934) (-34.6917, -46.2427) (-34.3358, -46.4452) knots 0 0 0 1 1 1
  spline S161 degree 2 poles (-34.3358, -46.4452) (-34.0387, -46.6182) (-33.6632, -46.6182) knots 0 0 0 1 1 1
  spline S162 degree 2 poles (-33.6632, -46.6182) (-33.2617, -46.6182) (-32.9743, -46.4256) knots 0 0 0 1 1 1
  spline S163 degree 2 poles (-32.9743, -46.4256) (-32.6413, -46.2068) (-32.6413, -45.8248) knots 0 0 0 1 1 1
  spline S164 degree 2 poles (-32.6413, -45.8248) (-32.6413, -45.4102) (-33.0592, -45.2273) knots 0 0 0 1 1 1
  spline S165 degree 2 poles (-33.0592, -45.2273) (-33.2062, -45.162) (-33.6567, -45.087) knots 0 0 0 1 1 1
  spline S166 degree 2 poles (-33.6567, -45.087) (-34.1954, -44.9988) (-34.4534, -44.8388) knots 0 0 0 1 1 1
  spline S167 degree 2 poles (-34.4534, -44.8388) (-34.8354, -44.6103) (-34.8354, -44.1532) knots 0 0 0 1 1 1
  spline S168 degree 2 poles (-34.8354, -44.1532) (-34.8354, -43.7092) (-34.4729, -43.4349) knots 0 0 0 1 1 1
  spline S169 degree 2 poles (-34.4729, -43.4349) (-34.1465, -43.19) (-33.6828, -43.19) knots 0 0 0 1 1 1
  spline S170 degree 2 poles (-33.6828, -43.19) (-33.1572, -43.19) (-32.7752, -43.5231) knots 0 0 0 1 1 1
  line L93 (-32.7752, -43.5231) -> (-32.7752, -43.4382)
  spline S171 degree 2 poles (-32.7752, -43.4382) (-32.7752, -43.2717) (-32.6479, -43.2717) knots 0 0 0 1 1 1
  spline S172 degree 2 poles (-32.6479, -43.2717) (-32.5238, -43.2717) (-32.5238, -43.4382) knots 0 0 0 1 1 1
  line L94 (-32.5238, -43.4382) -> (-32.5238, -44.0781)
  spline S173 degree 2 poles (-32.5238, -44.0781) (-32.5238, -44.2446) (-32.6479, -44.2446) knots 0 0 0 1 1 1
  spline S174 degree 2 poles (-32.6479, -44.2446) (-32.7654, -44.2446) (-32.7752, -44.0911) knots 0 0 0 1 1 1
  spline S175 degree 2 poles (-32.7752, -44.0911) (-32.7948, -43.7875) (-33.0886, -43.6014) knots 0 0 0 1 1 1
  spline S176 degree 2 poles (-33.0886, -43.6014) (-33.3498, -43.4414) (-33.6763, -43.4414) knots 0 0 0 1 1 1
  spline S177 degree 2 poles (-33.6763, -43.4414) (-34.0322, -43.4414) (-34.2901, -43.6177) knots 0 0 0 1 1 1
  spline S178 degree 2 poles (-34.2901, -43.6177) (-34.584, -43.8202) (-34.584, -44.1597) knots 0 0 0 1 1 1
  spline S179 degree 2 poles (-34.584, -44.1597) (-34.584, -44.4634) (-34.3326, -44.6299) knots 0 0 0 1 1 1
  spline S180 degree 2 poles (-34.3326, -44.6299) (-34.1269, -44.767) (-33.6241, -44.8519) knots 0 0 0 1 1 1
  spline S181 degree 2 poles (-33.6241, -44.8519) (-33.1082, -44.9368) (-32.9188, -45.0217) knots 0 0 0 1 1 1
  spline S182 degree 2 poles (-32.9188, -45.0217) (-32.3899, -45.26) (-32.3899, -45.8314) knots 0 0 0 1 1 1
  spline S183 degree 2 poles (-28.7169, -46.6443) (-28.7169, -46.7717) (-28.8867, -46.7717) knots 0 0 0 1 1 1
  line L95 (-28.8867, -46.7717) -> (-31.1133, -46.7717)
  spline S184 degree 2 poles (-31.1133, -46.7717) (-31.2799, -46.7717) (-31.2799, -46.6443) knots 0 0 0 1 1 1
  spline S185 degree 2 poles (-31.2799, -46.6443) (-31.2799, -46.5203) (-31.1133, -46.5203) knots 0 0 0 1 1 1
  line L96 (-31.1133, -46.5203) -> (-30.1241, -46.5203)
  line L97 (-30.1241, -46.5203) -> (-30.1241, -43.2717)
  line L98 (-30.1241, -43.2717) -> (-30.8489, -43.2717)
  spline S186 degree 2 poles (-30.8489, -43.2717) (-31.0187, -43.2717) (-31.0187, -43.1443) knots 0 0 0 1 1 1
  spline S187 degree 2 poles (-31.0187, -43.1443) (-31.0187, -43.017) (-30.8489, -43.017) knots 0 0 0 1 1 1
  line L99 (-30.8489, -43.017) -> (-29.8727, -43.017)
  line L100 (-29.8727, -43.017) -> (-29.8727, -46.5203)
  line L101 (-29.8727, -46.5203) -> (-28.8867, -46.5203)
  spline S188 degree 2 poles (-28.8867, -46.5203) (-28.7169, -46.5203) (-28.7169, -46.6443) knots 0 0 0 1 1 1
  spline S189 degree 2 poles (-24.8414, -46.6443) (-24.8414, -46.7717) (-25.0112, -46.7717) knots 0 0 0 1 1 1
  line L102 (-25.0112, -46.7717) -> (-25.6021, -46.7717)
  line L103 (-25.6021, -46.7717) -> (-25.6021, -46.4092)
  spline S190 degree 2 poles (-25.6021, -46.4092) (-26.1507, -46.8696) (-26.771, -46.8696) knots 0 0 0 1 1 1
  spline S191 degree 2 poles (-26.771, -46.8696) (-27.166, -46.8696) (-27.4305, -46.677) knots 0 0 0 1 1 1
  spline S192 degree 2 poles (-27.4305, -46.677) (-27.7309, -46.4615) (-27.7309, -46.0795) knots 0 0 0 1 1 1
  spline S193 degree 2 poles (-27.7309, -46.0795) (-27.7309, -45.6159) (-27.2836, -45.3677) knots 0 0 0 1 1 1
  spline S194 degree 2 poles (-27.2836, -45.3677) (-26.9212, -45.1718) (-26.4184, -45.1718) knots 0 0 0 1 1 1
  spline S195 degree 2 poles (-26.4184, -45.1718) (-26.0592, -45.1718) (-25.6021, -45.2633) knots 0 0 0 1 1 1
  line L104 (-25.6021, -45.2633) -> (-25.6021, -44.8584)
  spline S196 degree 2 poles (-25.6021, -44.8584) (-25.6021, -44.5907) (-25.8666, -44.4536) knots 0 0 0 1 1 1
  spline S197 degree 2 poles (-25.8666, -44.4536) (-26.0756, -44.3458) (-26.3661, -44.3458) knots 0 0 0 1 1 1
  spline S198 degree 2 poles (-26.3661, -44.3458) (-26.6567, -44.3458) (-27.1889, -44.5156) knots 0 0 0 1 1 1
  spline S199 degree 2 poles (-27.1889, -44.5156) (-27.2803, -44.545) (-27.3097, -44.545) knots 0 0 0 1 1 1
  spline S200 degree 2 poles (-27.3097, -44.545) (-27.4272, -44.545) (-27.4272, -44.4209) knots 0 0 0 1 1 1
  spline S201 degree 2 poles (-27.4272, -44.4209) (-27.4272, -44.3687) (-27.3979, -44.3393) knots 0 0 0 1 1 1
  spline S202 degree 2 poles (-27.3979, -44.3393) (-27.3554, -44.2936) (-27.0583, -44.2152) knots 0 0 0 1 1 1
  spline S203 degree 2 poles (-27.0583, -44.2152) (-26.5882, -44.0911) (-26.3531, -44.0911) knots 0 0 0 1 1 1
  spline S204 degree 2 poles (-26.3531, -44.0911) (-25.9678, -44.0911) (-25.6805, -44.2773) knots 0 0 0 1 1 1
  spline S205 degree 2 poles (-25.6805, -44.2773) (-25.3475, -44.4895) (-25.3475, -44.8584) knots 0 0 0 1 1 1
  line L105 (-25.3475, -44.8584) -> (-25.3475, -46.5203)
  line L106 (-25.3475, -46.5203) -> (-25.0112, -46.5203)
  spline S206 degree 2 poles (-25.0112, -46.5203) (-24.8414, -46.5203) (-24.8414, -46.6443) knots 0 0 0 1 1 1
  line L107 (-25.6021, -46.073) -> (-25.6021, -45.5212)
  spline S207 degree 2 poles (-25.6021, -45.5212) (-25.945, -45.4232) (-26.3923, -45.4232) knots 0 0 0 1 1 1
  spline S208 degree 2 poles (-26.3923, -45.4232) (-26.9342, -45.4232) (-27.2477, -45.6583) knots 0 0 0 1 1 1
  spline S209 degree 2 poles (-27.2477, -45.6583) (-27.4795, -45.8346) (-27.4795, -46.0795) knots 0 0 0 1 1 1
  spline S210 degree 2 poles (-27.4795, -46.0795) (-27.4795, -46.3537) (-27.2575, -46.4941) knots 0 0 0 1 1 1
  spline S211 degree 2 poles (-27.2575, -46.4941) (-27.0714, -46.6182) (-26.784, -46.6182) knots 0 0 0 1 1 1
  spline S212 degree 2 poles (-26.784, -46.6182) (-26.1702, -46.6182) (-25.6021, -46.073) knots 0 0 0 1 1 1
  spline S213 degree 2 poles (-21.1651, -46.6443) (-21.1651, -46.7717) (-21.3316, -46.7717) knots 0 0 0 1 1 1
  line L108 (-21.3316, -46.7717) -> (-22.0042, -46.7717)
  spline S214 degree 2 poles (-22.0042, -46.7717) (-22.174, -46.7717) (-22.174, -46.6443) knots 0 0 0 1 1 1
  spline S215 degree 2 poles (-22.174, -46.6443) (-22.174, -46.5203) (-22.0042, -46.5203) knots 0 0 0 1 1 1
  line L109 (-22.0042, -46.5203) -> (-21.7952, -46.5203)
  line L110 (-21.7952, -46.5203) -> (-21.7952, -44.9792)
  spline S216 degree 2 poles (-21.7952, -44.9792) (-21.7952, -44.6854) (-22.0107, -44.5091) knots 0 0 0 1 1 1
  spline S217 degree 2 poles (-22.0107, -44.5091) (-22.2099, -44.3458) (-22.5103, -44.3458) knots 0 0 0 1 1 1
  spline S218 degree 2 poles (-22.5103, -44.3458) (-22.8139, -44.3458) (-23.0522, -44.5221) knots 0 0 0 1 1 1
  spline S219 degree 2 poles (-23.0522, -44.5221) (-23.1894, -44.6233) (-23.4604, -44.9433) knots 0 0 0 1 1 1
  line L111 (-23.4604, -44.9433) -> (-23.4604, -46.5203)
  line L112 (-23.4604, -46.5203) -> (-23.1763, -46.5203)
  spline S220 degree 2 poles (-23.1763, -46.5203) (-23.0098, -46.5203) (-23.0098, -46.6443) knots 0 0 0 1 1 1
  spline S221 degree 2 poles (-23.0098, -46.6443) (-23.0098, -46.7717) (-23.1763, -46.7717) knots 0 0 0 1 1 1
  line L113 (-23.1763, -46.7717) -> (-23.9958, -46.7717)
  spline S222 degree 2 poles (-23.9958, -46.7717) (-24.1623, -46.7717) (-24.1623, -46.6443) knots 0 0 0 1 1 1
  spline S223 degree 2 poles (-24.1623, -46.6443) (-24.1623, -46.5203) (-23.9958, -46.5203) knots 0 0 0 1 1 1
  line L114 (-23.9958, -46.5203) -> (-23.7118, -46.5203)
  line L115 (-23.7118, -46.5203) -> (-23.7118, -44.4372)
  line L116 (-23.7118, -44.4372) -> (-23.924, -44.4372)
  spline S224 degree 2 poles (-23.924, -44.4372) (-24.0905, -44.4372) (-24.0905, -44.3099) knots 0 0 0 1 1 1
  spline S225 degree 2 poles (-24.0905, -44.3099) (-24.0905, -44.1826) (-23.924, -44.1826) knots 0 0 0 1 1 1
  line L117 (-23.924, -44.1826) -> (-23.4604, -44.1826)
  line L118 (-23.4604, -44.1826) -> (-23.4604, -44.5613)
  spline S226 degree 2 poles (-23.4604, -44.5613) (-22.9967, -44.0911) (-22.507, -44.0911) knots 0 0 0 1 1 1
  spline S227 degree 2 poles (-22.507, -44.0911) (-21.952, -44.0911) (-21.6777, -44.5091) knots 0 0 0 1 1 1
  spline S228 degree 2 poles (-21.6777, -44.5091) (-21.5438, -44.718) (-21.5438, -44.9368) knots 0 0 0 1 1 1
  line L119 (-21.5438, -44.9368) -> (-21.5438, -46.5203)
  line L120 (-21.5438, -46.5203) -> (-21.3316, -46.5203)
  spline S229 degree 2 poles (-21.3316, -46.5203) (-21.1651, -46.5203) (-21.1651, -46.6443) knots 0 0 0 1 1 1
  spline S230 degree 2 poles (-17.6814, -46.6443) (-17.6814, -46.7717) (-17.8512, -46.7717) knots 0 0 0 1 1 1
  line L121 (-17.8512, -46.7717) -> (-20.0779, -46.7717)
  spline S231 degree 2 poles (-20.0779, -46.7717) (-20.2444, -46.7717) (-20.2444, -46.6443) knots 0 0 0 1 1 1
  spline S232 degree 2 poles (-20.2444, -46.6443) (-20.2444, -46.5203) (-20.0779, -46.5203) knots 0 0 0 1 1 1
  line L122 (-20.0779, -46.5203) -> (-19.0886, -46.5203)
  line L123 (-19.0886, -46.5203) -> (-19.0886, -44.4372)
  line L124 (-19.0886, -44.4372) -> (-19.8232, -44.4372)
  spline S233 degree 2 poles (-19.8232, -44.4372) (-19.993, -44.4372) (-19.993, -44.3099) knots 0 0 0 1 1 1
  spline S234 degree 2 poles (-19.993, -44.3099) (-19.993, -44.1826) (-19.8232, -44.1826) knots 0 0 0 1 1 1
  line L125 (-19.8232, -44.1826) -> (-18.8372, -44.1826)
  line L126 (-18.8372, -44.1826) -> (-18.8372, -46.5203)
  line L127 (-18.8372, -46.5203) -> (-17.8512, -46.5203)
  spline S235 degree 2 poles (-17.8512, -46.5203) (-17.6814, -46.5203) (-17.6814, -46.6443) knots 0 0 0 1 1 1
  line L128 (-18.8438, -43.5426) -> (-19.216, -43.5426)
  line L129 (-19.216, -43.5426) -> (-19.216, -42.8929)
  line L130 (-19.216, -42.8929) -> (-18.8438, -42.8929)
  line L131 (-18.8438, -42.8929) -> (-18.8438, -43.5426)
  spline S236 degree 2 poles (-13.8125, -46.6443) (-13.8125, -46.7717) (-13.979, -46.7717) knots 0 0 0 1 1 1
  line L132 (-13.979, -46.7717) -> (-14.6516, -46.7717)
  spline S237 degree 2 poles (-14.6516, -46.7717) (-14.8214, -46.7717) (-14.8214, -46.6443) knots 0 0 0 1 1 1
  spline S238 degree 2 poles (-14.8214, -46.6443) (-14.8214, -46.5203) (-14.6516, -46.5203) knots 0 0 0 1 1 1
  line L133 (-14.6516, -46.5203) -> (-14.4426, -46.5203)
  line L134 (-14.4426, -46.5203) -> (-14.4426, -44.9792)
  spline S239 degree 2 poles (-14.4426, -44.9792) (-14.4426, -44.6854) (-14.6581, -44.5091) knots 0 0 0 1 1 1
  spline S240 degree 2 poles (-14.6581, -44.5091) (-14.8573, -44.3458) (-15.1577, -44.3458) knots 0 0 0 1 1 1
  spline S241 degree 2 poles (-15.1577, -44.3458) (-15.4613, -44.3458) (-15.6996, -44.5221) knots 0 0 0 1 1 1
  spline S242 degree 2 poles (-15.6996, -44.5221) (-15.8368, -44.6233) (-16.1077, -44.9433) knots 0 0 0 1 1 1
  line L135 (-16.1077, -44.9433) -> (-16.1077, -46.5203)
  line L136 (-16.1077, -46.5203) -> (-15.8237, -46.5203)
  spline S243 degree 2 poles (-15.8237, -46.5203) (-15.6572, -46.5203) (-15.6572, -46.6443) knots 0 0 0 1 1 1
  spline S244 degree 2 poles (-15.6572, -46.6443) (-15.6572, -46.7717) (-15.8237, -46.7717) knots 0 0 0 1 1 1
  line L137 (-15.8237, -46.7717) -> (-16.6432, -46.7717)
  spline S245 degree 2 poles (-16.6432, -46.7717) (-16.8097, -46.7717) (-16.8097, -46.6443) knots 0 0 0 1 1 1
  spline S246 degree 2 poles (-16.8097, -46.6443) (-16.8097, -46.5203) (-16.6432, -46.5203) knots 0 0 0 1 1 1
  line L138 (-16.6432, -46.5203) -> (-16.3591, -46.5203)
  line L139 (-16.3591, -46.5203) -> (-16.3591, -44.4372)
  line L140 (-16.3591, -44.4372) -> (-16.5714, -44.4372)
  spline S247 degree 2 poles (-16.5714, -44.4372) (-16.7379, -44.4372) (-16.7379, -44.3099) knots 0 0 0 1 1 1
  spline S248 degree 2 poles (-16.7379, -44.3099) (-16.7379, -44.1826) (-16.5714, -44.1826) knots 0 0 0 1 1 1
  line L141 (-16.5714, -44.1826) -> (-16.1077, -44.1826)
  line L142 (-16.1077, -44.1826) -> (-16.1077, -44.5613)
  spline S249 degree 2 poles (-16.1077, -44.5613) (-15.6441, -44.0911) (-15.1544, -44.0911) knots 0 0 0 1 1 1
  spline S250 degree 2 poles (-15.1544, -44.0911) (-14.5993, -44.0911) (-14.3251, -44.5091) knots 0 0 0 1 1 1
  spline S251 degree 2 poles (-14.3251, -44.5091) (-14.1912, -44.718) (-14.1912, -44.9368) knots 0 0 0 1 1 1
  line L143 (-14.1912, -44.9368) -> (-14.1912, -46.5203)
  line L144 (-14.1912, -46.5203) -> (-13.979, -46.5203)
  spline S252 degree 2 poles (-13.979, -46.5203) (-13.8125, -46.5203) (-13.8125, -46.6443) knots 0 0 0 1 1 1
  spline S253 degree 2 poles (-10.1362, -46.6443) (-10.1362, -46.7717) (-10.306, -46.7717) knots 0 0 0 1 1 1
  line L145 (-10.306, -46.7717) -> (-10.8969, -46.7717)
  line L146 (-10.8969, -46.7717) -> (-10.8969, -46.4092)
  spline S254 degree 2 poles (-10.8969, -46.4092) (-11.4454, -46.8696) (-12.0658, -46.8696) knots 0 0 0 1 1 1
  spline S255 degree 2 poles (-12.0658, -46.8696) (-12.4608, -46.8696) (-12.7253, -46.677) knots 0 0 0 1 1 1
  spline S256 degree 2 poles (-12.7253, -46.677) (-13.0257, -46.4615) (-13.0257, -46.0795) knots 0 0 0 1 1 1
  spline S257 degree 2 poles (-13.0257, -46.0795) (-13.0257, -45.6159) (-12.5784, -45.3677) knots 0 0 0 1 1 1
  spline S258 degree 2 poles (-12.5784, -45.3677) (-12.216, -45.1718) (-11.7132, -45.1718) knots 0 0 0 1 1 1
  spline S259 degree 2 poles (-11.7132, -45.1718) (-11.354, -45.1718) (-10.8969, -45.2633) knots 0 0 0 1 1 1
  line L147 (-10.8969, -45.2633) -> (-10.8969, -44.8584)
  spline S260 degree 2 poles (-10.8969, -44.8584) (-10.8969, -44.5907) (-11.1614, -44.4536) knots 0 0 0 1 1 1
  spline S261 degree 2 poles (-11.1614, -44.4536) (-11.3703, -44.3458) (-11.6609, -44.3458) knots 0 0 0 1 1 1
  spline S262 degree 2 poles (-11.6609, -44.3458) (-11.9515, -44.3458) (-12.4837, -44.5156) knots 0 0 0 1 1 1
  spline S263 degree 2 poles (-12.4837, -44.5156) (-12.5751, -44.545) (-12.6045, -44.545) knots 0 0 0 1 1 1
  spline S264 degree 2 poles (-12.6045, -44.545) (-12.722, -44.545) (-12.722, -44.4209) knots 0 0 0 1 1 1
  spline S265 degree 2 poles (-12.722, -44.4209) (-12.722, -44.3687) (-12.6926, -44.3393) knots 0 0 0 1 1 1
  spline S266 degree 2 poles (-12.6926, -44.3393) (-12.6502, -44.2936) (-12.3531, -44.2152) knots 0 0 0 1 1 1
  spline S267 degree 2 poles (-12.3531, -44.2152) (-11.8829, -44.0911) (-11.6479, -44.0911) knots 0 0 0 1 1 1
  spline S268 degree 2 poles (-11.6479, -44.0911) (-11.2626, -44.0911) (-10.9753, -44.2773) knots 0 0 0 1 1 1
  spline S269 degree 2 poles (-10.9753, -44.2773) (-10.6423, -44.4895) (-10.6423, -44.8584) knots 0 0 0 1 1 1
  line L148 (-10.6423, -44.8584) -> (-10.6423, -46.5203)
  line L149 (-10.6423, -46.5203) -> (-10.306, -46.5203)
  spline S270 degree 2 poles (-10.306, -46.5203) (-10.1362, -46.5203) (-10.1362, -46.6443) knots 0 0 0 1 1 1
  line L150 (-10.8969, -46.073) -> (-10.8969, -45.5212)
  spline S271 degree 2 poles (-10.8969, -45.5212) (-11.2397, -45.4232) (-11.687, -45.4232) knots 0 0 0 1 1 1
  spline S272 degree 2 poles (-11.687, -45.4232) (-12.229, -45.4232) (-12.5424, -45.6583) knots 0 0 0 1 1 1
  spline S273 degree 2 poles (-12.5424, -45.6583) (-12.7743, -45.8346) (-12.7743, -46.0795) knots 0 0 0 1 1 1
  spline S274 degree 2 poles (-12.7743, -46.0795) (-12.7743, -46.3537) (-12.5522, -46.4941) knots 0 0 0 1 1 1
  spline S275 degree 2 poles (-12.5522, -46.4941) (-12.3661, -46.6182) (-12.0788, -46.6182) knots 0 0 0 1 1 1
  spline S276 degree 2 poles (-12.0788, -46.6182) (-11.465, -46.6182) (-10.8969, -46.073) knots 0 0 0 1 1 1
  dimension "d2" = 6
  dimension "d3" = 0
  dimension "d35" = 40
  dimension "d36" = 10
  dimension "d37" = 10
  dimension "d38" = 6
  constraints: 2 other
  measures "d35" distance of L2.start L2.end
  measures "d36" distance of L4.end L2.start
  measures "d37" distance between parallel lines of L1 L3
  measures "d38" distance between parallel lines of L0 L4
extrude "Extrusion6" cut sketch "Sketch6" against normal blind 0.1
equation "\"d22\" = d21"
body "Solid1"
